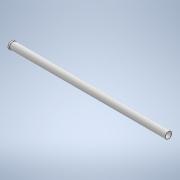
# Autodesk Inventor part: Lift.02.00.00.03
Saved by Autodesk Inventor 2021 (Build 250183000, 183)
## iProperties
Created: 2020-09-20
Part Number: Lift.02.00.00.03
Material: Типовые
Document SubType Name: Modeling
Designer: Kostya
Density: 1 g/cm^3
Appearance: По умолчанию
Author: Kostya
Autodesk Inventor part; units mm, degrees
ref_plane "YZ Plane" through (0, 0, 0) normal (1, 0, 0) x (0, 1, 0)
ref_plane "XZ Plane" through (0, 0, 0) normal (0, 1, 0) x (-1, 0, 0)
ref_plane "XY Plane" through (0, 0, 0) normal (0, 0, 1) x (1, 0, 0)
sketch "Эскиз1" plane through (0, 0, 0) normal (0, 0, 1) x (1, 0, 0)
  line L0 (0, 0) -> (-1408.8676, 0)
  line L1 (-3080, 0) -> (-3080, 72.5)
  line L2 (-3080, 72.5) -> (-3050, 72.5)
  line L3 (-3050, 72.5) -> (-3050, 67.5)
  line L4 (-3050, 67.5) -> (0, 67.5)
  line L5 (0, 67.5) -> (0, 0)
  line L6 (0, 57.5) -> (-3080, 57.5)
  dimension "d0" = 115
  dimension "d1" = 135
  dimension "d2" = 145
  dimension "d3" = 30
  dimension "d4" = 3080
  constraints: 14 end point, 5 perpendicular, 3 point on line, 1 horizontal, 1 vertical
  measures "d0" diameter of L6 L0
  measures "d1" diameter of L4 L0
  measures "d2" diameter of L2 L0
  measures "d3" distance of L1.end L2.end
  measures "d4" distance between parallel lines of L5 L1
revolve "Вращение1" add sketch "Эскиз1" angle 360 about axis through (0, 0, 0) along (-1, 0, 0)
